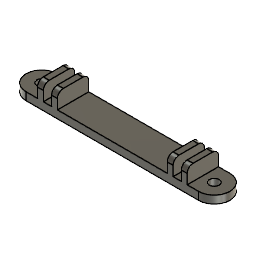
Shooter Mount (Autodesk Fusion 360 design; units mm, degrees)
Autodesk Fusion 360 part; units mm, degrees
sketch "Sketch1" plane through (0, 0, 0) normal (0, 0, 1) x (1, 0, 0)
  line L0 (52, 8) -> (-52, 8)
  line L1 (-52, 8) -> (-52, -8)
  line L2 (-52, -8) -> (52, -8)
  line L3 (52, -8) -> (52, 8)
  line L4 (52, 8) -> (-52, -8) construction
  line L5 (-52, 8) -> (52, -8) construction
  circle A0 centre (-44, 0) radius 2.5
  line L6 (-38.2, 8) -> (-38.2, -8)
  line L7 (-35.2, 8) -> (-35.2, -8)
  line L8 (-31, 8) -> (-31, -8)
  line L9 (-28, 8) -> (-28, -8)
  line L10 (0, 1.75) -> (0, 22.5)
  line L11 (28, 8) -> (28, -8)
  line L12 (31, 8) -> (31, -8)
  line L13 (35.2, 8) -> (35.2, -8)
  line L14 (38.2, 8) -> (38.2, -8)
  circle A1 centre (44, 0) radius 2.5
  dimension "d1" = 104
  dimension "d2" = 16
  dimension "d3" = 5
  dimension "d4" = 8
  dimension "d6" = 3
  dimension "d7" = 31
  dimension "d8" = 3
  dimension "d9" = 4.2
  constraint horizontal L0
  constraint perpendicular L0 L1
  constraint parallel L0 L2
  constraint parallel L1 L3
  constraint coincident L4 origin
  constraint coincident L5 origin
  constraint coincident L0 L6.start
  constraint coincident L2 L6.end
  constraint perpendicular L2 L6
  constraint coincident L0 L7.start
  constraint coincident L2 L7.end
  constraint perpendicular L2 L7
  constraint coincident L0 L8.start
  constraint coincident L2 L8.end
  constraint perpendicular L2 L8
  constraint coincident L0 L9.start
  constraint coincident L2 L9.end
  constraint perpendicular L2 L9
  constraint horizontal origin A0.centre
  constraint symmetric A0 L10 A1
  constraint symmetric L6.start L10 L14.start
  constraint symmetric L6.end L10 L14.end
  constraint symmetric L7.start L10 L13.start
  constraint symmetric L7.end L10 L13.end
  constraint symmetric L8.start L10 L12.start
  constraint symmetric L8.end L10 L12.end
  constraint symmetric L9.start L10 L11.start
  constraint symmetric L9.end L10 L11.end
  measures "d1" distance of L1.end L2.end
  measures "d2" distance of L0.end L1.end
  measures "d3" diameter of A0
  measures "d4" distance of L1 A0.centre
  measures "d6" distance of L6 L7
  measures "d7" distance of origin L8
  measures "d8" distance of L8 L9
  measures "d9" distance of L7 L8
extrude "Extrude1" add sketch "Sketch1" along normal blind 4
extrude "Extrude2" add sketch "Sketch1" along normal blind 12 contours L0 L2 L13 L14 | L0 L2 L11 L12 | L0 L2 L8 L9 | L0 L2 L6 L7
fillet "Fillet1" radius 8 4 edges at (-52, -8, 2) (-52, 8, 2) (52, 8, 2) (52, -8, 2)
fillet "Fillet1" radius 3 8 edges at (-36.7, -8, 12) (-36.7, 8, 12) (-29.5, -8, 12) (-29.5, 8, 12) (29.5, 8, 12) (29.5, -8, 12) (36.7, -8, 12) (36.7, 8, 12)
